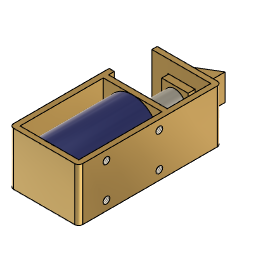
The vault v47 (Autodesk Fusion 360 archive; units mm, degrees)
design "Solenoid"
Autodesk Fusion 360 part; units mm, degrees
sketch "Sketch1" plane through (0, 0, 0) normal (0, 0, 1) x (1, 0, 0)
  line L0 (-13.1, 18.85) -> (-11.1, 18.85)
  line L1 (-11.1, 18.85) -> (-11.1, -18.85)
  line L2 (-11.1, -18.85) -> (-13.1, -18.85)
  line L3 (-13.1, -18.85) -> (-13.1, 18.85)
  line L4 (-13.1, -18.85) -> (13.1, -18.85)
  line L5 (13.1, -18.85) -> (13.1, -16.85)
  line L6 (13.1, -16.85) -> (-13.1, -16.85)
  line L7 (-13.1, -16.85) -> (-13.1, -18.85)
  line L8 (13.1, -18.85) -> (11.1, -18.85)
  line L9 (11.1, -18.85) -> (11.1, 35.15)
  line L10 (11.1, 35.15) -> (13.1, 35.15)
  line L11 (13.1, 35.15) -> (13.1, -18.85)
  line L12 (13.1, 35.15) -> (-11.2, 35.15)
  line L13 (-11.2, 35.15) -> (-11.2, 33.15)
  line L14 (-11.2, 33.15) -> (13.1, 33.15)
  line L15 (13.1, 33.15) -> (13.1, 35.15)
  line L16 (-11.1, 16.65) -> (11.1, 16.65)
  line L17 (11.1, 16.65) -> (11.1, 14.65)
  line L18 (11.1, 14.65) -> (-11.1, 14.65)
  line L19 (-11.1, 14.65) -> (-11.1, 16.65)
  dimension "d1" = 2
  dimension "d2" = 2
  dimension "d3" = 2
  dimension "d4" = 2
  dimension "d5" = 2
  dimension "d6" = 26.2
  dimension "d7" = 37.7
  dimension "d8" = 35.5
  dimension "d9" = 54
  dimension "d10" = 24.3
  dimension "d36" = 13.1
  dimension "d37" = 18.85
  constraint horizontal L0
  constraint vertical L1
  constraint horizontal L2
  constraint vertical L3
  constraint horizontal L4
  constraint vertical L5
  constraint horizontal L6
  constraint vertical L7
  constraint horizontal L8
  constraint vertical L9
  constraint horizontal L10
  constraint vertical L11
  constraint horizontal L12
  constraint vertical L13
  constraint horizontal L14
  constraint vertical L15
  constraint horizontal L16
  constraint vertical L17
  constraint horizontal L18
  constraint vertical L19
  constraint coincident L9 L17.end
  constraint coincident L1 L16.start
  measures "d1" distance of L1 L3
  measures "d2" distance of L4 L6
  measures "d3" distance of L16 L18
  measures "d4" distance of L9 L11
  measures "d5" distance of L12 L14
  measures "d6" distance of L3 L11
  measures "d7" distance of L0.start L4
  measures "d8" distance of L4 L16
  measures "d9" distance of L4 L12
  measures "d10" distance of L10.end L12.end
  measures "d36" distance of origin L3
  measures "d37" distance of origin L4
extrude "Extrude1" add sketch "Sketch1" along normal mid plane 20 contours L0 L1 L3 L6 L19 | L1 L2 L3 L4 L6 L7 | L1 L9 L16 L17 L18 L19 | L1 L4 L6 L9 | L6 L9 L11 L14 L17 | L4 L5 L6 L8 L9 L11 | L9 L12 L13 L14 | L9 L10 L11 L12 L14 L15
sketch "Sketch2" plane through (0, 14.65, 0) normal (0, -1, 0) x (1, 0, 0)
  line L0 (-11.1, -10) -> (11.1, -10)
  line L1 (11.1, -10) -> (11.1, 10)
  line L2 (11.1, 10) -> (-11.1, 10)
  line L3 (-11.1, 10) -> (-11.1, -10)
  circle A0 centre (0, 0) radius 10
  dimension "d13" = 20
  dimension "d14" = 10
  dimension "d15" = 22.2
  dimension "d16" = 11.1
  constraint tangent L2 A0
  measures "d13" distance of L0 L2
  measures "d14" distance of L2 A0.centre
  measures "d15" distance of L1 L3
  measures "d16" distance of L3 A0.centre
extrude "Extrude2" add sketch "Sketch2" along normal blind 32 contours A0
fillet "Fillet1" radius 1.5 3 edges at (-13.1, -18.85, 0) (13.1, -18.85, 0) (13.1, 35.15, 0)
sketch "Sketch3" plane through (0, 16.65, 0) normal (0, 1, 0) x (-1, 0, 0)
  line L0 (-11.1, -10) -> (11.1, -10)
  line L1 (11.1, -10) -> (11.1, 10)
  line L2 (11.1, 10) -> (-11.1, 10)
  line L3 (-11.1, 10) -> (-11.1, -10)
  line L4 (-11.6, -10) -> (-13.1, -10)
  line L5 (-11.6, -10) -> (11.6, -10)
  line L6 (13.1, -10) -> (11.6, -10)
  line L7 (-13.1, -10) -> (-13.1, 10)
  line L8 (-13.1, 10) -> (-11.6, 10)
  line L9 (11.6, 10) -> (13.1, 10)
  line L10 (13.1, 10) -> (13.1, -10)
  line L11 (11.6, 10) -> (-11.6, 10)
  circle A0 centre (0, 0) radius 4
  arc A1 (0, -10) -> (0, 10) centre (0, 0) ccw
  arc A2 (0, 10) -> (0, -10) centre (0, 0) ccw
  arc A3 (0, -10) -> (0, 10) centre (0, 0) ccw
  arc A4 (0, 10) -> (0, -10) centre (0, 0) ccw
  dimension "d20" = 8
  constraint concentric A0 A1
  measures "d20" diameter of A0
extrude "Extrude3" add sketch "Sketch3" along normal blind 15 contours A0
sketch "Sketch5" plane through (0, 35.15, 0) normal (0, 1, 0) x (-1, 0, 0)
  line L0 (-11.6, 10) -> (-11.6, -10)
  line L1 (-11.6, -10) -> (11.2, -10)
  line L2 (11.2, -10) -> (11.2, 10)
  line L3 (11.2, 10) -> (-11.6, 10)
  circle A0 centre (0, 0) radius 4
  circle A1 centre (0, 0) radius 4
  line L4 (5.15, 5.15) -> (-5.15, 5.15)
  line L5 (-5.15, 5.15) -> (-5.15, -5.15)
  line L6 (-5.15, -5.15) -> (5.15, -5.15)
  line L7 (5.15, -5.15) -> (5.15, 5.15)
  line L8 (5.15, 5.15) -> (-5.15, -5.15) construction
  line L9 (-5.15, 5.15) -> (5.15, -5.15) construction
  dimension "d30" = 10.3
  dimension "d31" = 10.3
  constraint perpendicular L4 L5
  constraint parallel L4 L6
  constraint parallel L5 L7
  constraint horizontal L4
  constraint coincident L8 A0.centre
  constraint coincident L9 A0.centre
  constraint coincident A0.centre A1.centre
  measures "d30" distance of L5.end L6.end
  measures "d31" distance of L4.end L5.end
extrude "Extrude5" cut sketch "Sketch5" against normal blind 4 contours A0 A1 | L4 L5 L6 L7
sketch "Sketch4" plane through (0, 0, 0) normal (0, 0, 1) x (1, 0, 0)
  line L0 (-5, 30.65) -> (5, 30.65)
  line L1 (5, 30.65) -> (5, 44.65)
  line L2 (5, 44.65) -> (-5, 44.65)
  line L3 (-5, 44.65) -> (-5, 30.65)
  line L4 (5, 44.65) -> (-5, 38.65)
  line L5 (-11.1, 16.65) -> (11.1, 16.65)
  dimension "d23" = 10
  dimension "d26" = 14
  dimension "d27" = 8
  dimension "d35" = 28
  dimension "d38" = 5
  constraint horizontal L0
  constraint vertical L1
  constraint horizontal L2
  constraint vertical L3
  constraint coincident L3 L4.end
  measures "d23" distance of L1.end L2.end
  measures "d26" distance of L0.end L2
  measures "d27" distance of L0 L4.end
  measures "d35" distance of L1.end L5
  measures "d38" distance of origin L3
extrude "Extrude4" add sketch "Sketch4" along normal mid plane 10 contours L0 L1 L3 L4
sketch "Sketch6" plane through (13.1, 0, 0) normal (1, 0, 0) x (0, 1, 0)
  line L0 (33.65, -10) -> (33.65, 10)
  line L1 (33.65, 10) -> (-17.35, 10)
  line L2 (-17.35, 10) -> (-17.35, -10)
  line L3 (-17.35, -10) -> (33.65, -10)
  line L4 (35.15, -10) -> (35.15, 10)
  point P0 (-8.35, 6.5)
  point P1 (11.65, 6.5)
  point P2 (11.65, -6.5)
  point P3 (-8.35, -6.5)
  dimension "d39" = 13
  dimension "d40" = 6.5
  dimension "d41" = 20
  dimension "d42" = 23.5
  dimension "d46" = 13
  constraint horizontal P0 P1
  constraint vertical P1 P2
  constraint vertical P0 P3
  measures "d39" distance of P0 P3
  measures "d40" vertical distance of origin P0
  measures "d41" distance of P0 P1
  measures "d42" distance of P1 L4
  measures "d46" distance of P1 P2
hole "Hole1" at (13.1, 11.65, 6.5) at (13.1, 11.65, -6.5) at (13.1, -8.35, -6.5) at (13.1, -8.35, 6.5) direction (-1, 0, 0) diameter 2.529 depth 2 tip angle 180
thread "Thread1" "ISO Metric profile 3.0 M3x0.5 6H" major diameter 3.086 minor diameter 2.529 pitch 0.5 angle 60 resizes the face on face at (11.7667, 11.7759, 5.2418) on face at (11.7667, 11.7759, -7.7582) on face at (11.7667, -8.2241, -7.7582) on face at (11.7667, -8.2241, 5.2418)
equation "d2 = d1"
equation "d3 = d1"
equation "d4 = d1"
equation "d5 = d1"
equation "d36 = d6 / 2"
equation "d37 = d7 / 2"
equation "d38 = d23 / 2"
equation "d40 = d39 / 2"
equation "d46 = d39"
